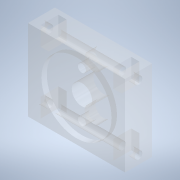
# Autodesk Inventor part: motorfogo
Saved by Autodesk Inventor 2022 (Build 260153000, 153)
## iProperties
Created: 2021-10-06
Part Number: motorfogo
Material: PC/ABS Plastic
Document SubType Name: Modeling
Designer: Varga Tamás
Density: 0.357273 g/cm^3
Appearance: Smooth - White
Mass: 2.92193 g
Surface Area: 49.2665 cm^2
Volume: 8.17844 cm^3
Author: Varga Tamás
Autodesk Inventor part; units mm, degrees
ref_plane "YZ Plane" through (0, 0, 0) normal (1, 0, 0) x (0, 1, 0)
ref_plane "XZ Plane" through (0, 0, 0) normal (0, 1, 0) x (-1, 0, 0)
ref_plane "XY Plane" through (0, 0, 0) normal (0, 0, 1) x (1, 0, 0)
sketch "Sketch1" plane through (0, 0, 0) normal (0, 0, 1) x (1, 0, 0)
  circle A0 centre (0, 0) radius 15
  circle A1 centre (0, 0) radius 8.5
  line L0 (0, 8.5) -> (0, -8.5)
  circle A2 centre (0, 0) radius 3.75
  line L1 (18, -15) -> (-18, -15)
  line L2 (-18, -15) -> (-18, 15)
  line L3 (-18, 15) -> (18, 15)
  line L4 (18, 15) -> (18, -15)
  point P0 (0, 15)
  point P1 (0, -15)
  dimension "d0" = 30
  dimension "d1" = 17
  dimension "d2" = 7.5
  dimension "d15" = 30
  dimension "d16" = 36
  dimension "d17" = 18
  dimension "d18" = 15
  constraints: 10 end point, 5 coincident, 3 centre point, 2 parallel, 2 point on circle, 1 horizontal, 1 perpendicular, 1 vertical
  measures "d0" diameter of A0
  measures "d1" diameter of A1
  measures "d2" diameter of A2
  measures "d15" distance of L3.end L1.start
  measures "d16" distance of L1.start L1.end
  measures "d17" distance from line of A0.centre L2
  measures "d18" distance from line of A0.centre L3
extrude "Extrusion1" add sketch "Sketch1" along normal blind 10 contours A0 | A1 L0 A2 | L0 A2 A1
hole "Hole1" at (0, 8.5, 0) at (0, -8.5, 0) direction (0, 0, 1) diameter 3 end through all
sketch "Sketch2" plane through (0, 0, 10) normal (0, 0, 1) x (1, 0, 0)
  circle A0 centre (0, 0) radius 13
  dimension "d12" = 26
  constraints: 1 centre point, 1 coincident
  measures "d12" diameter of A0
extrude "Extrusion2" cut sketch "Sketch2" against normal blind 2
extrude "Extrusion3" add sketch "Sketch1" along normal blind 10 contours A0 L3 L4 L1 | A0 L1 L2 L3
sketch "Sketch4" plane through (-18, -15, 0) normal (-1, 0, 0) x (0, 0, 1)
  line L0 (5, 27) -> (5, 3)
  line L1 (0, 30) -> (0, 0) projected
  line L2 (0, 0) -> (10, 0) projected
  line L3 (0, 30) -> (10, 30) projected
  point P0 (0, 15)
  dimension "d21" = 5
  dimension "d22" = 24
  dimension "d23" = 3
  dimension "d24" = 3
  constraints: 2 coincident, 2 end point
  measures "d21" distance between parallel lines of L1 L0
  measures "d22" distance of L0.start L0.end
  measures "d23" distance from line of L2 L0.end
  measures "d24" distance from line of L3 L0.start
hole "Hole2" at (-18, 12, 5) at (-18, -12, 5) direction (1, 0, 0) diameter 2.8 end through all
sketch "Sketch5" plane through (18, -15, 0) normal (1, 0, 0) x (0, 0, -1)
  circle A0 centre (-5, 27) radius 1.4 projected
  line L0 (-5, 27) -> (-5, 3)
  line L1 (0, 5) -> (-8, 5) projected
  point P0 (0, 15)
  dimension "d32" = 24
  constraints: 2 coincident, 2 end point, 1 perpendicular
  measures "d32" distance of L0.start L0.end
hole "Hole3" at (18, 12, 5) at (18, -12, 5) direction (-1, 0, 0) diameter 2.8 depth 8
sketch "Sketch6" plane through (-18, -15, 0) normal (0, -1, 0) x (1, 0, 0)
  line L0 (3, 8.3) -> (6, 8.3)
  line L1 (6, 8.3) -> (6, 1.7)
  line L2 (6, 1.7) -> (3, 1.7)
  line L3 (3, 1.7) -> (3, 8.3)
  line L4 (0, 10) -> (36, 10) projected
  line L5 (0, 0) -> (0, 10) projected
  line L6 (33, 8.3) -> (30, 8.3)
  line L7 (30, 8.3) -> (30, 1.7)
  line L8 (30, 1.7) -> (33, 1.7)
  line L9 (33, 1.7) -> (33, 8.3)
  line L10 (36, 0) -> (36, 10) projected
  line L11 (0, 0) -> (36, 0) projected
  point P0 (18, 0)
  dimension "d40" = 6.6
  dimension "d41" = 3
  dimension "d42" = 1.7
  dimension "d43" = 3
  dimension "d44" = 3
  dimension "d45" = 3
  dimension "d46" = 6.6
  dimension "d47" = 1.7
  constraints: 16 end point, 4 parallel, 2 horizontal, 2 perpendicular
  measures "d40" distance of L0.end L1.end
  measures "d41" distance of L0.start L0.end
  measures "d42" distance between parallel lines of L4 L0
  measures "d43" distance between parallel lines of L5 L3
  measures "d44" distance of L6.start L6.end
  measures "d45" distance between parallel lines of L9 L10
  measures "d46" distance of L8.end L6.start
  measures "d47" distance between parallel lines of L11 L8
extrude "Extrusion4" cut sketch "Sketch6" against normal blind 7 contours L0 L1 L2 L3 | L9 L8 L7 L6
sketch "Sketch7" plane through (-18, 15, 0) normal (0, 1, 0) x (1, 0, 0)
  line L0 (33, -8.3) -> (30, -8.3)
  line L1 (30, -8.3) -> (30, -1.7)
  line L2 (30, -1.7) -> (33, -1.7)
  line L3 (33, -1.7) -> (33, -8.3)
  line L4 (3, -8.3) -> (6, -8.3)
  line L5 (6, -8.3) -> (6, -1.7)
  line L6 (6, -1.7) -> (3, -1.7)
  line L7 (3, -1.7) -> (3, -8.3)
  line L8 (0, 0) -> (0, -10) projected
  line L9 (36, 0) -> (36, -10) projected
  line L10 (36, 0) -> (0, 0) projected
  point P0 (18, 0)
  dimension "d50" = 3
  dimension "d51" = 3
  dimension "d52" = 3
  dimension "d53" = 3
  dimension "d54" = 1.7
  dimension "d55" = 1.7
  dimension "d56" = 6.6
  dimension "d57" = 6.6
  constraints: 16 end point, 4 parallel, 2 horizontal, 2 perpendicular
  measures "d50" distance of L0.start L0.end
  measures "d51" distance of L4.start L4.end
  measures "d52" distance between parallel lines of L7 L8
  measures "d53" distance between parallel lines of L9 L3
  measures "d54" distance between parallel lines of L10 L2
  measures "d55" distance between parallel lines of L10 L6
  measures "d56" distance of L4.end L5.end
  measures "d57" distance of L0.end L1.end
extrude "Extrusion5" cut sketch "Sketch7" against normal blind 7
sketch "Sketch8" plane through (0, 0, 0) normal (0, 0, -1) x (-1, 0, 0)
  circle A0 centre (0, -8.5) radius 1.5 projected
  circle A1 centre (0, 8.5) radius 1.5 projected
  circle A2 centre (0, -8.5) radius 1.5 projected
  circle A3 centre (0, -8.5) radius 3
  circle A4 centre (0, 8.5) radius 1.5 projected
  circle A5 centre (0, 8.5) radius 3
  point P0 (0, 0)
  dimension "d60" = 6
  dimension "d61" = 6
  constraints: 2 centre point, 2 coincident
  measures "d60" diameter of A3
  measures "d61" diameter of A5
extrude "Extrusion6" cut sketch "Sketch8" against normal blind 4
body "Solid1"
